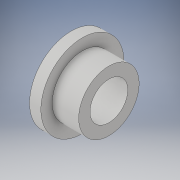
# Autodesk Inventor part: Parts_GEF
Saved by Autodesk Inventor 2019.4 (Build 234330000, 330)
## iProperties
Created: 2019-07-22
Part Number: Parts_GEF
Material: 一般
Document SubType Name: Modeling
Designer: Koki Shinjo
Mass: 0.220304 g
Surface Area: 3.69137 cm^2
Volume: 0.220304 cm^3
Density: 1 g/cm^3
Appearance: 既定
Author: Koki Shinjo
Autodesk Inventor part; units mm, degrees
ref_plane "YZ Plane" through (0, 0, 0) normal (1, 0, 0) x (0, 1, 0)
ref_plane "XZ Plane" through (0, 0, 0) normal (0, 1, 0) x (-1, 0, 0)
ref_plane "XY Plane" through (0, 0, 0) normal (0, 0, 1) x (1, 0, 0)
sketch "スケッチ1" plane through (0, 0, 0) normal (0, 0, 1) x (1, 0, 0)
  line L0 (0, 2.5) -> (0, 5.5)
  line L1 (0, 5.5) -> (1.5, 5.5)
  line L2 (1.5, 5.5) -> (1.5, 4)
  line L3 (1.5, 4) -> (5, 4)
  line L4 (5, 4) -> (5, 2.5)
  line L5 (5, 2.5) -> (0, 2.5)
  line L6 (-1, 0) -> (6, 0) projected
  point P0 (0, 0)
  dimension "d0" = 2.5
  dimension "d1" = 4
  dimension "d2" = 5
  dimension "d3" = 1.5
  dimension "d4" = 5.5
  constraints: 12 end point, 5 perpendicular, 1 vertical, 1 vertical alignment
  measures "d0" distance from line of point (0, 0) L5
  measures "d1" distance from line of point (0, 0) L3
  measures "d2" distance of L4.end L0.start
  measures "d3" distance of L0.end L1.end
  measures "d4" distance from line of point (0, 0) L1
revolve "回転1" add sketch "スケッチ1" angle 360 about axis through (-10, 0, 0) along (1, 0, 0)
